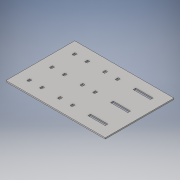
# Autodesk Inventor part: panel
Saved by Autodesk Inventor 2016 (Build 200138000, 138)
## iProperties
Created: 2016-07-20
Part Number: panel
Material: Generic
Document SubType Name: Modeling
Designer: Zuhra Abdurashidova
Density: 1 g/cm^3
Appearance: Default
Author: Zuhra Abdurashidova
Autodesk Inventor part; units mm, degrees
ref_plane "YZ Plane" through (0, 0, 0) normal (1, 0, 0) x (0, 1, 0)
ref_plane "XZ Plane" through (0, 0, 0) normal (0, 1, 0) x (-1, 0, 0)
ref_plane "XY Plane" through (0, 0, 0) normal (0, 0, 1) x (1, 0, 0)
sketch "Sketch1" plane through (0, 0, 0) normal (0, 1, 0) x (-1, 0, 0)
  line L0 (0, 0) -> (-250, 0)
  line L1 (-250, 0) -> (-250, -173)
  line L2 (-250, -173) -> (0, -173)
  line L3 (0, -173) -> (0, 0)
  line L4 (-32, -147) -> (-32, -140)
  line L5 (-26, -140) -> (-26, -147)
  arc A0 (-32, -147) -> (-26, -147) centre (-29, -140.6754) ccw
  arc A1 (-26, -140) -> (-32, -140) centre (-29, -146.3246) ccw
  line L6 (-64, -147) -> (-64, -140)
  line L7 (-58, -140) -> (-58, -147)
  arc A2 (-64, -147) -> (-58, -147) centre (-61, -140.6754) ccw
  arc A3 (-58, -140) -> (-64, -140) centre (-61, -146.3246) ccw
  line L8 (-109, -147) -> (-109, -140)
  line L9 (-103, -140) -> (-103, -147)
  arc A4 (-109, -147) -> (-103, -147) centre (-106, -140.6754) ccw
  arc A5 (-103, -140) -> (-109, -140) centre (-106, -146.3246) ccw
  line L10 (-141, -147) -> (-141, -140)
  line L11 (-135, -140) -> (-135, -147)
  arc A6 (-141, -147) -> (-135, -147) centre (-138, -140.6754) ccw
  arc A7 (-135, -140) -> (-141, -140) centre (-138, -146.3246) ccw
  line L12 (-32, -90) -> (-32, -83)
  line L13 (-26, -83) -> (-26, -90)
  arc A8 (-32, -90) -> (-26, -90) centre (-29, -83.6754) ccw
  arc A9 (-26, -83) -> (-32, -83) centre (-29, -89.3246) ccw
  line L14 (-32, -33) -> (-32, -26)
  line L15 (-26, -26) -> (-26, -33)
  arc A10 (-32, -33) -> (-26, -33) centre (-29, -26.6754) ccw
  arc A11 (-26, -26) -> (-32, -26) centre (-29, -32.3246) ccw
  line L16 (-64, -90) -> (-64, -83)
  line L17 (-58, -83) -> (-58, -90)
  arc A12 (-64, -90) -> (-58, -90) centre (-61, -83.6754) ccw
  arc A13 (-58, -83) -> (-64, -83) centre (-61, -89.3246) ccw
  line L18 (-109, -90) -> (-109, -83)
  line L19 (-103, -83) -> (-103, -90)
  arc A14 (-109, -90) -> (-103, -90) centre (-106, -83.6754) ccw
  arc A15 (-103, -83) -> (-109, -83) centre (-106, -89.3246) ccw
  line L20 (-141, -90) -> (-141, -83)
  line L21 (-135, -83) -> (-135, -90)
  arc A16 (-141, -90) -> (-135, -90) centre (-138, -83.6754) ccw
  arc A17 (-135, -83) -> (-141, -83) centre (-138, -89.3246) ccw
  line L22 (-58, -26) -> (-58, -33)
  arc A18 (-58, -26) -> (-64, -26) centre (-61, -32.3246) ccw
  line L23 (-64, -33) -> (-64, -26)
  arc A19 (-64, -33) -> (-58, -33) centre (-61, -26.6754) ccw
  line L24 (-103, -26) -> (-103, -33)
  arc A20 (-103, -26) -> (-109, -26) centre (-106, -32.3246) ccw
  line L25 (-109, -33) -> (-109, -26)
  arc A21 (-109, -33) -> (-103, -33) centre (-106, -26.6754) ccw
  line L26 (-135, -26) -> (-135, -33)
  arc A22 (-135, -26) -> (-141, -26) centre (-138, -32.3246) ccw
  line L27 (-141, -33) -> (-141, -26)
  arc A23 (-141, -33) -> (-135, -33) centre (-138, -26.6754) ccw
  line L28 (-180, -147) -> (-224, -147)
  line L29 (-224, -147) -> (-224, -140)
  line L30 (-224, -140) -> (-180, -140)
  line L31 (-180, -140) -> (-180, -147)
  line L32 (-180, -90) -> (-224, -90)
  line L33 (-224, -90) -> (-224, -83)
  line L34 (-224, -83) -> (-180, -83)
  line L35 (-180, -83) -> (-180, -90)
  line L36 (-180, -33) -> (-224, -33)
  line L37 (-224, -33) -> (-224, -26)
  line L38 (-224, -26) -> (-180, -26)
  line L39 (-180, -26) -> (-180, -33)
  dimension "d0" = 250
  dimension "d1" = 173
  dimension "d2" = 7
  dimension "d3" = 7
  dimension "d5" = 6
  dimension "d6" = 7
  dimension "d7" = 26
  dimension "d8" = 26
  dimension "d9" = 7
  dimension "d10" = 7
  dimension "d11" = 6
  dimension "d12" = 7
  dimension "d13" = 58
  dimension "d14" = 26
  dimension "d15" = 8.3509
  dimension "d16" = 7
  dimension "d17" = 7
  dimension "d18" = 6
  dimension "d19" = 7
  dimension "d20" = 103
  dimension "d21" = 26
  dimension "d22" = 7
  dimension "d23" = 7
  dimension "d24" = 6
  dimension "d25" = 7
  dimension "d26" = 135
  dimension "d27" = 26
  dimension "d28" = 7
  dimension "d29" = 7
  dimension "d30" = 6
  dimension "d31" = 7
  dimension "d32" = 8.3509
  dimension "d33" = 83
  dimension "d34" = 26
  dimension "d35" = 7
  dimension "d36" = 7
  dimension "d37" = 6
  dimension "d38" = 7
  dimension "d39" = 8.3509
  dimension "d40" = 140
  dimension "d41" = 26
  dimension "d42" = 7
  dimension "d43" = 7
  dimension "d44" = 6
  dimension "d45" = 7
  dimension "d46" = 8.3509
  dimension "d47" = 83
  dimension "d48" = 58
  dimension "d49" = 7
  dimension "d50" = 7
  dimension "d51" = 6
  dimension "d52" = 7
  dimension "d53" = 8.3509
  dimension "d54" = 83
  dimension "d55" = 103
  dimension "d56" = 7
  dimension "d57" = 7
  dimension "d58" = 6
  dimension "d59" = 7
  dimension "d60" = 8.3509
  dimension "d61" = 83
  dimension "d62" = 135
  dimension "d63" = 7
  dimension "d64" = 7
  constraints: 80 end point, 48 point on circle, 24 centre point, 20 parallel, 4 horizontal, 4 perpendicular
  measures "d0" distance of L1.end L2.end
  measures "d1" distance of L0.end L1.end
  measures "d2" radius of A0
  measures "d3" radius of A1
  measures "d5" distance between parallel lines of L4 L5
  measures "d6" distance of L5.start L5.end
  measures "d7" distance between parallel lines of L5 L3
  measures "d8" distance from line of L2 L5.end
  measures "d9" radius of A2
  measures "d10" radius of A3
  measures "d11" distance between parallel lines of L6 L7
  measures "d12" distance of L7.start L7.end
  measures "d13" distance between parallel lines of L3 L7
  measures "d14" distance from line of L7.end L2
  measures "d16" radius of A4
  measures "d17" radius of A5
  measures "d18" distance between parallel lines of L8 L9
  measures "d19" distance of L9.start L9.end
  measures "d20" distance between parallel lines of L3 L9
  measures "d21" distance from line of L2 L9.end
  measures "d22" radius of A6
  measures "d23" radius of A7
  measures "d24" distance between parallel lines of L10 L11
  measures "d25" distance of L11.start L11.end
  measures "d26" distance between parallel lines of L3 L11
  measures "d27" distance from line of L2 L11.end
  measures "d28" radius of A8
  measures "d29" radius of A9
  measures "d30" distance between parallel lines of L12 L13
  measures "d31" distance of L13.start L13.end
  measures "d33" distance from line of L2 L13.end
  measures "d34" distance between parallel lines of L3 L13
  measures "d35" radius of A10
  measures "d36" radius of A11
  measures "d37" distance between parallel lines of L14 L15
  measures "d38" distance of L15.start L15.end
  measures "d40" distance from line of L2 L15.end
  measures "d41" distance between parallel lines of L3 L15
  measures "d42" radius of A12
  measures "d43" radius of A13
  measures "d44" distance between parallel lines of L16 L17
  measures "d45" distance of L17.start L17.end
  measures "d47" distance from line of L2 L17.end
  measures "d48" distance between parallel lines of L3 L17
  measures "d49" radius of A14
  measures "d50" radius of A15
  measures "d51" distance between parallel lines of L18 L19
  measures "d52" distance of L19.start L19.end
  measures "d54" distance from line of L2 L19.end
  measures "d55" distance between parallel lines of L3 L19
  measures "d56" radius of A16
  measures "d57" radius of A17
  measures "d58" distance between parallel lines of L20 L21
  measures "d59" distance of L21.start L21.end
  measures "d61" distance from line of L2 L21.end
  measures "d62" distance between parallel lines of L3 L21
  measures "d63" radius of A19
  measures "d64" radius of A18
extrude "Extrusion1" add sketch "Sketch1" along normal blind 3.25 draft 3.2
body "Solid1"
